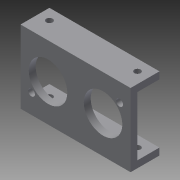
# Autodesk Inventor part: ping_bracket
Saved by Autodesk Inventor 2015 (Build 190159000, 159)
## iProperties
Created: 2014-10-29
Part Number: ping_bracket
Material: Generic
Document SubType Name: Modeling
Designer: Colin
Density: 1 g/cm^3
Appearance: Default
Author: Colin
Autodesk Inventor part; units mm, degrees
ref_plane "YZ Plane" through (0, 0, 0) normal (1, 0, 0) x (0, 1, 0)
ref_plane "XZ Plane" through (0, 0, 0) normal (0, 1, 0) x (-1, 0, 0)
ref_plane "XY Plane" through (0, 0, 0) normal (0, 0, 1) x (1, 0, 0)
sketch "Sketch1" plane through (0, 0, 0) normal (1, 0, 0) x (0, 1, 0)
  line L0 (0, 0) -> (30.48, 0)
  line L1 (30.48, -3.175) -> (3.175, -3.175)
  line L2 (3.175, -3.175) -> (3.175, -13.335)
  line L3 (3.175, -13.335) -> (0, -13.335)
  line L4 (0, -13.335) -> (0, 0)
  line L5 (30.48, 0) -> (33.655, 0)
  line L6 (33.655, 0) -> (33.655, -13.335)
  line L7 (33.655, -13.335) -> (30.48, -13.335)
  line L8 (30.48, -13.335) -> (30.48, -3.175)
  dimension "d0" = 3.175
  dimension "d1" = 30.48
  dimension "d33" = 13.335
  dimension "d34" = 3.175
  dimension "d36" = 3.175
  dimension "d37" = 13.335
  constraints: 18 end point, 4 perpendicular, 2 horizontal, 2 parallel
  measures "d0" distance of L2.end L3.end
  measures "d1" distance of L0.start L0.end
  measures "d33" distance of L3.end L0.start
  measures "d34" distance of L0.end L1.start
  measures "d36" distance of L6.end L7.end
  measures "d37" distance of L5.end L6.end
extrude "Extrusion1" add sketch "Sketch1" along normal blind 50.8
sketch "Sketch3" plane through (0, 0, 0) normal (0, 0, 1) x (1, 0, 0)
  line L0 (0, 30.48) -> (50.8, 30.48) projected
  line L1 (25.4, 30.48) -> (25.4, 3.175) construction
  line L2 (0, 3.175) -> (50.8, 3.175) projected
  circle A0 centre (12.7, 17.145) radius 8.89
  circle A1 centre (38.1, 17.145) radius 8.89
  line L3 (0, 0) -> (0, 30.48) projected
  line L4 (0, 27.813) -> (50.8, 27.813) construction
  line L5 (0, 6.477) -> (50.8, 6.477) construction
  line L6 (2.54, 27.813) -> (2.54, 6.477) construction
  line L7 (48.26, 27.813) -> (48.26, 6.477) construction
  circle A2 centre (5.08, 9.017) radius 1.5875
  circle A3 centre (45.72, 25.273) radius 1.5875
  dimension "d6" = 13.335
  dimension "d7" = 17.78
  dimension "d8" = 12.7
  dimension "d13" = 10.668
  dimension "d14" = 10.668
  dimension "d15" = 10.16
  dimension "d16" = 10.16
  dimension "d17" = 3.175
  dimension "d19" = 2.54
  dimension "d20" = 3.175
  dimension "d21" = 2.54
  dimension "d25" = 2.54
  dimension "d26" = 2.54
  constraints: 10 end point, 6 point on line, 4 centre point, 2 horizontal, 2 midpoint, 2 perpendicular, 1 symmetric about line, 1 other
  measures "d6" distance from line of L0 A0.centre
  measures "d7" diameter of A0
  measures "d8" distance from line of L1 A0.centre
  measures "d13" distance from line of A1.centre L5
  measures "d14" distance from line of A1.centre L4
  measures "d15" distance from line of A0.centre L6
  measures "d16" distance from line of A1.centre L7
  measures "d17" diameter of A2
  measures "d19" distance from line of L6 A2.centre
  measures "d20" diameter of A3
  measures "d21" distance from line of L7 A3.centre
  measures "d25" distance from line of L5 A2.centre
  measures "d26" distance from line of L4 A3.centre
extrude "Extrusion2" cut sketch "Sketch3" against normal through all
sketch "Sketch4" plane through (0, 3.175, -3.175) normal (0, 1, 0) x (1, 0, 0)
  circle A0 centre (5.08, 5.08) radius 1.4772
  circle A1 centre (45.72, 5.08) radius 1.451
  line L0 (50.8, 10.16) -> (50.8, 0) projected
  line L1 (0, 0) -> (50.8, 0) projected
  line L2 (0, 10.16) -> (50.8, 10.16) projected
  line L3 (0, 0) -> (0, 10.16) projected
  point P0 (0, -3.175)
  dimension "d27" = 5.08
  dimension "d29" = 5.08
  dimension "d30" = 5.08
  dimension "d35" = 5.08
  constraints: 2 centre point
  measures "d27" distance from line of L0 A1.centre
  measures "d29" distance from line of L2 A0.centre
  measures "d30" distance from line of A0.centre L3
  measures "d35" distance from line of L2 A1.centre
extrude "Extrusion3" cut sketch "Sketch4" along normal through all both and the other way through all contours A0 | A1
body "Solid1"
